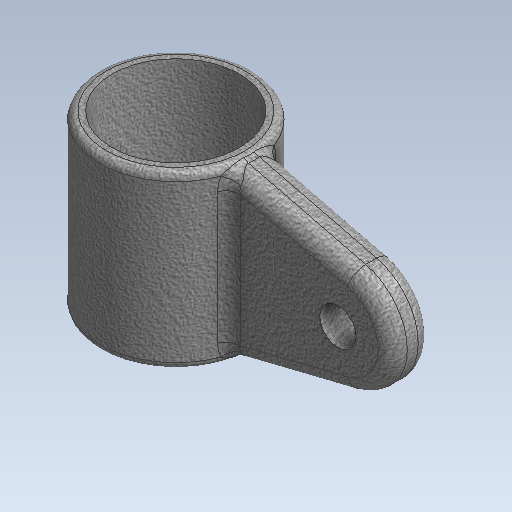
# Autodesk Inventor part: LM50-6
Saved by Autodesk Inventor 2021 (Build 250183000, 183)
## iProperties
Created: 2020-04-23
Part Number: LM50-6
Material: Aluminium Cast
Document SubType Name: Modeling
Designer: Hannah
Density: 2.7 g/cm^3
Appearance: Aluminum Cast
Mass: 120 g
Surface Area: 153.918 cm^2
Volume: 34.1913 cm^3
Vendor: Kee Systems
Description: male single swivel socket
Catalog Web Link: https://keesystems.com/store/fittings/kee-lite/lm50-male-single-swivel-socket-member.html
Size: 6
Author: Hannah
Revision Number: -
Autodesk Inventor part; units mm, degrees
ref_plane "YZ Plane" through (0, 0, 0) normal (1, 0, 0) x (0, 1, 0)
ref_plane "XZ Plane" through (0, 0, 0) normal (0, 1, 0) x (-1, 0, 0)
ref_plane "XY Plane" through (0, 0, 0) normal (0, 0, 1) x (1, 0, 0)
sketch "Sketch2" plane through (0, 0, 0) normal (0, 1, 0) x (-1, 0, 0)
  circle A0 centre (0, 0) radius 17.5
  circle A1 centre (0, 0) radius 21
  dimension "d5" = 35
  dimension "d6" = 42
  constraints: 2 centre point, 2 coincident
  measures "d5" diameter of A0
  measures "d6" diameter of A1
extrude "Extrusion2" add sketch "Sketch2" along normal mid plane 47 contours A0 | A1
extrude "Extrusion3" cut sketch "Sketch2" along normal through all both and the other way through all contours A0
hole "Hole1" at (0, 0, 0) direction (-1, 0, 0) diameter 8.376 end through all thread size "M10x1.5" class "6H" standard "ISO Metric profile"
sketch "Sketch3" plane through (0, 0, 0) normal (0, 0, 1) x (1, 0, 0)
  circle A0 centre (50, 0) radius 5
  arc A1 (53.6052, -14.5603) -> (53.6052, 14.5603) centre (50, 0) ccw
  line L0 (17.5, 23.5) -> (53.6052, 14.5603)
  line L1 (53.6052, -14.5603) -> (17.5, -23.5)
  line L2 (0, -35) -> (0, 35) projected
  line L3 (17.5, -23.5) -> (17.5, 23.5) projected
  point P0 (0, 0)
  dimension "d36" = 10
  dimension "d37" = 15
  dimension "d40" = 50
  constraints: 4 end point, 2 centre point, 2 point on circle, 2 tangent, 1 coincident, 1 equal length
  measures "d36" diameter of A0
  measures "d37" radius of A1
  measures "d40" distance from line of L2 A0.centre
extrude "Extrusion5" add sketch "Sketch3" along normal mid plane 11
fillet "Fillet2" radius 4 6 edges at (65, 0, 5.5) (36.9361, -18.6876, 5.5) (36.9361, 18.6876, 5.5) (65, 0, -5.5) (36.9361, -18.6876, -5.5) (36.9361, 18.6876, -5.5)
fillet "Fillet2" radius 2 2 edges at (21, 23.5, 0) (21, -23.5, 0)
fillet "Fillet3" radius 4 12 edges at (20.267, 0, 5.5) (20.3377, 20.159, 5.2322) (20.5521, 22.4081, 3.0824) (20.5691, 22.7401, 0) (20.5521, 22.4082, -3.0824) (20.3377, 20.159, -5.2322) (20.267, 0, -5.5) (20.3377, -20.159, -5.2322) (20.5521, -22.4082, -3.0824) (20.5691, -22.7401, 0) (20.5521, -22.4081, 3.0824) (20.3377, -20.159, 5.2322)
body "Solid1"
